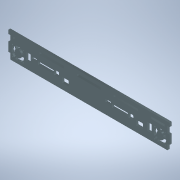
# Autodesk Inventor part: case top back
Saved by Autodesk Inventor 2022 (Build 260153000, 153)
## iProperties
Created: 2021-05-28
Part Number: case top back
Material: Lead
Document SubType Name: Modeling
Designer: benka
Density: 11.34 g/cm^3
Appearance: Lead
Author: benka
Autodesk Inventor part; units mm, degrees
ref_plane "YZ Plane" through (0, 0, 0) normal (1, 0, 0) x (0, 1, 0)
ref_plane "XZ Plane" through (0, 0, 0) normal (0, 1, 0) x (-1, 0, 0)
ref_plane "XY Plane" through (0, 0, 0) normal (0, 0, 1) x (1, 0, 0)
sketch "Sketch1" plane through (0, 0, 0) normal (0, 0, 1) x (1, 0, 0)
  line L0 (-48.3596, 9.6174) -> (-48.3596, -8.4526)
  line L1 (-48.3596, -8.4526) -> (-58.0817, -8.4526)
  line L2 (-58.0817, 9.6174) -> (-58.0817, -8.4526)
  line L3 (-45.5464, 0.7392) -> (-34.5464, 0.7392)
  line L4 (-33.5464, 1.7392) -> (-33.5464, 6.2392)
  line L5 (-34.5464, 7.2392) -> (-45.5464, 7.2392)
  line L6 (-46.5464, 6.2392) -> (-46.5464, 1.7392)
  line L7 (-30.7466, -2.0842) -> (3.2534, -2.0842)
  line L8 (4.2534, -1.0842) -> (4.2534, 3.9158)
  line L9 (-31.7466, 3.9158) -> (-31.7466, -1.0842)
  circle A0 centre (-88.9996, -15.383) radius 1.5
  circle A1 centre (-64.9996, -15.383) radius 1.5
  circle A2 centre (-64.9996, 8.617) radius 1.5
  circle A3 centre (-88.9996, 8.617) radius 1.5
  arc A4 (-82.1595, 3.0543) -> (-82.1595, -9.8202) centre (-76.9996, -3.383) ccw
  arc A5 (-79.9944, -11.0702) -> (-68.8448, -4.633) centre (-76.9996, -3.383) ccw
  arc A6 (-68.8448, -2.133) -> (-79.9944, 4.3043) centre (-76.9996, -3.383) ccw
  arc A7 (-82.0034, -16.8856) -> (-62.804, -5.8009) centre (-76.9996, -3.383) ccw
  arc A8 (-63.7898, -2.133) -> (-62.804, -0.9651) centre (-63.7898, -1.133) ccw
  arc A9 (-62.804, -0.9651) -> (-82.0034, 10.1197) centre (-76.9996, -3.383) ccw
  arc A10 (-82.0034, 10.1197) -> (-82.5219, 8.682) centre (-81.6559, 9.182) ccw
  line L10 (-82.5219, 8.682) -> (-79.9944, 4.3043)
  line L11 (-82.1595, 3.0543) -> (-84.687, 7.432)
  arc A11 (-84.687, 7.432) -> (-86.1913, 7.7018) centre (-85.553, 6.932) ccw
  arc A12 (-86.1913, 7.7018) -> (-86.1913, -14.4677) centre (-76.9996, -3.383) ccw
  arc A13 (-86.1913, -14.4677) -> (-84.687, -14.1979) centre (-85.553, -13.6979) ccw
  line L12 (-84.687, -14.1979) -> (-82.1595, -9.8202)
  arc A14 (-82.5219, -15.4479) -> (-82.0034, -16.8856) centre (-81.6559, -15.9479) ccw
  line L13 (-79.9944, -11.0702) -> (-82.5219, -15.4479)
  line L14 (-63.7898, -4.633) -> (-68.8448, -4.633)
  arc A15 (-62.804, -5.8009) -> (-63.7898, -4.633) centre (-63.7898, -5.633) ccw
  line L15 (-68.8448, -2.133) -> (-63.7898, -2.133)
  line L16 (-48.3596, 9.6174) -> (-58.0817, 9.6174)
  line L17 (3.2534, 4.9158) -> (-30.7466, 4.9158)
  arc A16 (-34.5464, 0.7392) -> (-33.5464, 1.7392) centre (-34.5464, 1.7392) ccw
  arc A17 (-33.5464, 6.2392) -> (-34.5464, 7.2392) centre (-34.5464, 6.2392) ccw
  arc A18 (-45.5464, 7.2392) -> (-46.5464, 6.2392) centre (-45.5464, 6.2392) ccw
  arc A19 (-46.5464, 1.7392) -> (-45.5464, 0.7392) centre (-45.5464, 1.7392) ccw
  arc A20 (-31.7466, -1.0842) -> (-30.7466, -2.0842) centre (-30.7466, -1.0842) ccw
  arc A21 (-30.7466, 4.9158) -> (-31.7466, 3.9158) centre (-30.7466, 3.9158) ccw
  arc A22 (4.2534, 3.9158) -> (3.2534, 4.9158) centre (3.2534, 3.9158) ccw
  arc A23 (3.2534, -2.0842) -> (4.2534, -1.0842) centre (3.2534, -1.0842) ccw
  line L18 (-93.9991, 32.6183) -> (267.0009, 32.6183)
  line L19 (216.5121, 9.6174) -> (226.4543, 9.6174)
  line L20 (226.4543, -8.4526) -> (216.5121, -8.4526)
  line L21 (216.5121, -8.4526) -> (216.5121, 9.6174)
  line L22 (226.4543, -8.4526) -> (226.4543, 9.6174)
  line L23 (206.4252, -9.0821) -> (206.4252, 0.4179)
  line L24 (205.4252, 1.4179) -> (192.4252, 1.4179)
  line L25 (192.4252, -10.0821) -> (205.4252, -10.0821)
  line L26 (137.2814, -2.0492) -> (171.2814, -2.0492)
  line L27 (172.2814, -1.0492) -> (172.2814, 3.9508)
  line L28 (184.4118, -2.8933) -> (184.4118, 5.6067)
  line L29 (191.4252, 0.4179) -> (191.4252, -9.0821)
  line L30 (174.6118, -3.8933) -> (183.4118, -3.8933)
  line L31 (136.2814, 3.9508) -> (136.2814, -1.0492)
  line L32 (134.4536, 1.7392) -> (134.4536, 6.2392)
  line L33 (122.4536, 0.7392) -> (133.4536, 0.7392)
  line L34 (133.4536, 7.2392) -> (122.4536, 7.2392)
  line L35 (121.4536, 6.2392) -> (121.4536, 1.7392)
  circle A24 centre (232.9975, -15.3839) radius 1.5
  circle A25 centre (256.9975, -15.3839) radius 1.5
  circle A26 centre (256.9975, 8.6161) radius 1.5
  circle A27 centre (232.9975, 8.6161) radius 1.5
  line L36 (239.4751, 8.6811) -> (242.0026, 4.3033)
  arc A28 (239.9936, 10.1188) -> (239.4751, 8.6811) centre (240.3411, 9.1811) ccw
  arc A29 (259.193, -0.966) -> (239.9936, 10.1188) centre (244.9975, -3.3839) ccw
  arc A30 (253.1522, -2.1339) -> (242.0026, 4.3033) centre (244.9975, -3.3839) ccw
  line L37 (253.1522, -2.1339) -> (258.2072, -2.1339)
  arc A31 (258.2072, -2.1339) -> (259.193, -0.966) centre (258.2072, -1.1339) ccw
  arc A32 (242.0029, -11.0712) -> (253.1525, -4.6339) centre (244.9977, -3.3839) ccw
  line L38 (237.31, -14.1989) -> (239.8375, -9.8211)
  arc A33 (235.8057, -14.4686) -> (237.31, -14.1989) centre (236.444, -13.6989) ccw
  arc A34 (235.8057, 7.7009) -> (235.8057, -14.4686) centre (244.9975, -3.3839) ccw
  arc A35 (239.8375, 3.0533) -> (239.8375, -9.8211) centre (244.9975, -3.3839) ccw
  line L39 (239.8375, 3.0533) -> (237.31, 7.4311)
  arc A36 (237.31, 7.4311) -> (235.8057, 7.7009) centre (236.444, 6.9311) ccw
  line L40 (173.6118, -2.8933) -> (173.6118, 5.6067)
  line L41 (174.6118, 6.6067) -> (183.4118, 6.6067)
  line L42 (171.2814, 4.9508) -> (137.2814, 4.9508)
  arc A37 (133.4536, 0.7392) -> (134.4536, 1.7392) centre (133.4536, 1.7392) ccw
  arc A38 (134.4536, 6.2392) -> (133.4536, 7.2392) centre (133.4536, 6.2392) ccw
  arc A39 (122.4536, 7.2392) -> (121.4536, 6.2392) centre (122.4536, 6.2392) ccw
  arc A40 (121.4536, 1.7392) -> (122.4536, 0.7392) centre (122.4536, 1.7392) ccw
  arc A41 (136.2814, -1.0492) -> (137.2814, -2.0492) centre (137.2814, -1.0492) ccw
  arc A42 (137.2814, 4.9508) -> (136.2814, 3.9508) centre (137.2814, 3.9508) ccw
  arc A43 (172.2814, 3.9508) -> (171.2814, 4.9508) centre (171.2814, 3.9508) ccw
  arc A44 (171.2814, -2.0492) -> (172.2814, -1.0492) centre (171.2814, -1.0492) ccw
  arc A45 (173.6118, -2.8933) -> (174.6118, -3.8933) centre (174.6118, -2.8933) ccw
  arc A46 (174.6118, 6.6067) -> (173.6118, 5.6067) centre (174.6118, 5.6067) ccw
  arc A47 (184.4118, 5.6067) -> (183.4118, 6.6067) centre (183.4118, 5.6067) ccw
  arc A48 (183.4118, -3.8933) -> (184.4118, -2.8933) centre (183.4118, -2.8933) ccw
  arc A49 (192.4252, 1.4179) -> (191.4252, 0.4179) centre (192.4252, 0.4179) ccw
  arc A50 (191.4252, -9.0821) -> (192.4252, -10.0821) centre (192.4252, -9.0821) ccw
  arc A51 (205.4252, -10.0821) -> (206.4252, -9.0821) centre (205.4252, -9.0821) ccw
  arc A52 (206.4252, 0.4179) -> (205.4252, 1.4179) centre (205.4252, 0.4179) ccw
  line L43 (242.0029, -11.0712) -> (239.4754, -15.4489)
  arc A53 (239.4754, -15.4489) -> (239.9936, -16.8864) centre (240.3414, -15.9489) ccw
  line L44 (258.2072, -4.6339) -> (253.1525, -4.6339)
  arc A54 (239.9936, -16.8864) -> (259.193, -5.8017) centre (244.9975, -3.3838) ccw
  arc A55 (259.193, -5.8017) -> (258.2072, -4.6339) centre (258.2072, -5.6339) ccw
  line L45 (267.0009, 32.6183) -> (267.0009, 24.6181) projected
  line L46 (267.0009, 24.6181) -> (262.0009, 24.6181) projected
  line L47 (262.0009, 24.6181) -> (262.0009, 9.6181) projected
  line L48 (267.0009, 9.6181) -> (262.0009, 9.6181) projected
  line L49 (267.0009, 9.6181) -> (267.0009, -10.3826) projected
  line L50 (267.0009, -10.3826) -> (262.0009, -10.3826) projected
  line L51 (262.0009, -10.3826) -> (262.0009, -23.3826)
  line L52 (-93.9991, 24.6181) -> (-98.9991, 24.6181) projected
  line L53 (-93.9991, 24.6181) -> (-93.9991, 9.6181) projected
  line L54 (-93.9991, 9.6181) -> (-98.9991, 9.6181) projected
  line L55 (-98.9991, 9.6181) -> (-98.9991, -10.3826) projected
  line L56 (-93.9991, -10.3826) -> (-98.9991, -10.3826) projected
  line L57 (-93.9991, -10.3826) -> (-93.9991, -23.3826)
  arc A56 (15.2717, -3.613) -> (16.2717, -2.613) centre (15.2717, -2.613) ccw
  arc A57 (16.2717, 5.887) -> (15.2717, 6.887) centre (15.2717, 5.887) ccw
  line L58 (5.4717, -2.613) -> (5.4717, 5.887)
  arc A58 (5.4717, -2.613) -> (6.4717, -3.613) centre (6.4717, -2.613) ccw
  arc A59 (6.4717, 6.887) -> (5.4717, 5.887) centre (6.4717, 5.887) ccw
  line L59 (6.4717, 6.887) -> (15.2717, 6.887)
  line L60 (6.4717, -3.613) -> (15.2717, -3.613)
  line L61 (23.4252, 0.4179) -> (23.4252, -9.0821)
  line L62 (37.4252, 1.4179) -> (24.4252, 1.4179)
  line L63 (24.4252, -10.0821) -> (37.4252, -10.0821)
  line L64 (38.4252, -9.0821) -> (38.4252, 0.4179)
  line L65 (16.2717, -2.613) -> (16.2717, 5.887)
  arc A60 (24.4252, 1.4179) -> (23.4252, 0.4179) centre (24.4252, 0.4179) ccw
  arc A61 (23.4252, -9.0821) -> (24.4252, -10.0821) centre (24.4252, -9.0821) ccw
  arc A62 (37.4252, -10.0821) -> (38.4252, -9.0821) centre (37.4252, -9.0821) ccw
  arc A63 (38.4252, 0.4179) -> (37.4252, 1.4179) centre (37.4252, 0.4179) ccw
  line L66 (-98.9991, 32.6183) -> (-98.9991, 24.6181) projected
  line L67 (-93.9991, 32.6183) -> (-98.9991, 32.6183) projected
  line L68 (-87.4991, 24.6174) -> (-57.4991, 24.6174) projected
  line L69 (-57.4991, 24.6174) -> (-57.4991, 19.6174) projected
  line L70 (-87.4991, 19.6174) -> (-57.4991, 19.6174) projected
  line L71 (-87.4991, 24.6174) -> (-87.4991, 19.6174) projected
  line L72 (-27.4991, 24.6174) -> (27.5009, 24.6174) projected
  line L73 (27.5009, 24.6174) -> (27.5009, 19.6174) projected
  line L74 (-27.4991, 19.6174) -> (27.5009, 19.6174) projected
  line L75 (-27.4991, 24.6174) -> (-27.4991, 19.6174) projected
  line L76 (57.5009, 24.6174) -> (110.5009, 24.6174) projected
  line L77 (110.5009, 24.6174) -> (110.5009, 19.6174) projected
  line L78 (57.5009, 19.6174) -> (110.5009, 19.6174) projected
  line L79 (57.5009, 24.6174) -> (57.5009, 19.6174) projected
  line L80 (140.5009, 24.6174) -> (195.5009, 24.6174) projected
  line L81 (195.5009, 24.6174) -> (195.5009, 19.6174) projected
  line L82 (140.5009, 19.6174) -> (195.5009, 19.6174) projected
  line L83 (140.5009, 24.6174) -> (140.5009, 19.6174) projected
  line L84 (225.5009, 24.6174) -> (255.5009, 24.6174) projected
  line L85 (255.5009, 24.6174) -> (255.5009, 19.6174) projected
  line L86 (225.5009, 19.6174) -> (255.5009, 19.6174) projected
  line L87 (225.5009, 24.6174) -> (225.5009, 19.6174) projected
  line L88 (-93.9991, -23.3826) -> (262.0009, -23.3826) projected
  point P0 (94.0004, -33.3808)
  point P1 (-46.5464, 0.7392)
  point P2 (-33.5464, 7.2392)
  point P3 (-33.5464, 0.7392)
  point P4 (-46.5464, 7.2392)
  point P5 (-31.7466, -2.0842)
  point P6 (4.2534, 4.9158)
  point P7 (4.2534, -2.0842)
  point P8 (-31.7466, 4.9158)
  point P9 (206.4252, 1.4179)
  point P10 (206.4252, -10.0821)
  point P11 (191.4252, 1.4179)
  point P12 (191.4252, -10.0821)
  point P13 (136.2814, -2.0492)
  point P14 (172.2814, -2.0492)
  point P15 (172.2814, 4.9508)
  point P16 (136.2814, 4.9508)
  point P17 (173.6118, -3.8933)
  point P18 (184.4118, 6.6067)
  point P19 (184.4118, -3.8933)
  point P20 (134.4536, 0.7392)
  point P21 (134.4536, 7.2392)
  point P22 (121.4536, 0.7392)
  point P23 (121.4536, 7.2392)
  point P24 (23.4252, 1.4179)
  point P25 (5.4717, -3.613)
  point P26 (16.2717, 6.887)
  point P27 (16.2717, -3.613)
  point P28 (23.4252, -10.0821)
  point P29 (38.4252, -10.0821)
  point P30 (38.4252, 1.4179)
  dimension "d53" = 6.5
  dimension "d54" = 13
  dimension "d56" = 36
  dimension "d59" = 1
  dimension "d60" = 7
  dimension "d65" = 6.5
  dimension "d66" = 13
  dimension "d67" = 36
  dimension "d68" = 10.5
  dimension "d69" = 10.8
  dimension "d70" = 1
  dimension "d71" = 7
  dimension "d72" = 11.5
  dimension "d73" = 15
  dimension "d78" = 10.5
  dimension "d79" = 10.8
  dimension "d80" = 11.5
  dimension "d81" = 15
  dimension "d85" = 13
  constraints: 112 point on circle, 110 end point, 64 centre point, 64 tangent, 61 point on line, 22 equal radius, 5 horizontal, 3 perpendicular, 2 vertical, 1 parallel
  measures "d53" distance between parallel lines of L5 L3
  measures "d54" distance between parallel lines of L4 L6
  measures "d56" distance between parallel lines of L9 L8
  measures "d59" radius of A16
  measures "d60" distance between parallel lines of L17 L7
  measures "d65" distance between parallel lines of L34 L33
  measures "d66" distance between parallel lines of L32 L35
  measures "d67" distance between parallel lines of L31 L27
  measures "d68" distance between parallel lines of L41 L30
  measures "d69" distance of point (173.612, -3.893) point (184.412, -3.893)
  measures "d70" radius of A37
  measures "d71" distance between parallel lines of L42 L26
  measures "d72" distance between parallel lines of L25 L24
  measures "d73" distance between parallel lines of L23 L29
  measures "d78" distance between parallel lines of L59 L60
  measures "d79" distance of point (5.472, -3.613) point (16.272, -3.613)
  measures "d80" distance between parallel lines of L63 L62
  measures "d81" distance between parallel lines of L64 L61
  measures "d85" distance of L56.start L57.end
extrude "Extrusion2" add sketch "Sketch1" along normal blind 5
body "Solid2"
